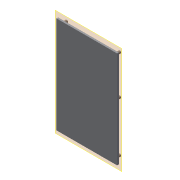
# Autodesk Inventor part: 200_Gearbox_conterplate
Saved by Autodesk Inventor 2019 (Build 230136000, 136)
## iProperties
Created: 2019-07-08
Part Number: 200_Gearbox_conterplate
Material: Generic
Document SubType Name: Modeling
Designer: diederichbenedict
Density: 1 g/cm^3
Appearance: Default
Author: diederichbenedict
Autodesk Inventor part; units mm, degrees
ref_plane "YZ Plane" through (0, 0, 0) normal (1, 0, 0) x (0, 1, 0)
ref_plane "XZ Plane" through (0, 0, 0) normal (0, 1, 0) x (-1, 0, 0)
ref_plane "XY Plane" through (0, 0, 0) normal (0, 0, 1) x (1, 0, 0)
ref_plane "Work Plane1" through (0, 0, 0) normal (0, 0, 1) x (1, 0, 0)
sketch "Sketch1" plane through (0, 0, 0) normal (0, 0, 1) x (1, 0, 0)
  circle A0 centre (-12.2447, -18.3325) radius 0.75 projected
  circle A1 centre (12.2447, 22.8412) radius 0.75 projected
  circle A2 centre (12.2447, 4.8925) radius 0.75 projected
  circle A3 centre (-12.2447, 4.8925) radius 0.75 projected
  circle A4 centre (12.2447, -18.3325) radius 0.75 projected
  circle A5 centre (-12.2447, 22.8412) radius 0.75 projected
  line L0 (-14, -20.0878) -> (14, -20.0878) projected
  line L1 (14, -20.0878) -> (14, 24.5965) projected
  line L2 (14, 24.5965) -> (8.6716, 24.5965) projected
  arc A6 (7.3084, 6.3656) -> (8.6716, 24.5965) centre (0, 16.0785) ccw projected
  line L3 (7.3084, 6.3656) -> (7.3084, 3.43) projected
  arc A7 (-7.3084, 3.43) -> (7.3084, 3.43) centre (0, -6.0878) ccw projected
  line L4 (-7.3084, 3.43) -> (-7.3084, 6.3656) projected
  arc A8 (-8.6716, 24.5965) -> (-7.3084, 6.3656) centre (0, 16.0785) ccw projected
  line L5 (-8.6716, 24.5965) -> (-14, 24.5965) projected
  line L6 (-14, 24.5965) -> (-14, -20.0878) projected
  line L7 (8.6716, 24.5965) -> (-8.6716, 24.5965)
  point P0 (0, 0)
  constraints: 2 end point, 1 horizontal
extrude "Extrusion1" add sketch "Sketch1" along normal blind 0.8 contours A0 | A1 | A2 | A3 | A4 | A5 | L6 L5 A8 L4 A7 L3 A6 L2 L1 L0 | L7 A6 L3 A7 L4 A8
sketch "Sketch2" plane through (0, 0, 0.8) normal (0, 0, 1) x (1, 0, 0)
  circle A0 centre (-12.2447, -18.3325) radius 0.75 construction
  circle A1 centre (12.2447, 22.8412) radius 0.75 construction
  circle A2 centre (12.2447, 4.8925) radius 0.75 construction
  circle A3 centre (-12.2447, 4.8925) radius 0.75 construction
  circle A4 centre (12.2447, -18.3325) radius 0.75 construction
  circle A5 centre (-12.2447, 22.8412) radius 0.75 construction
  circle A6 centre (0, -6.0878) radius 9.5 construction
  line L0 (14, -20.0878) -> (-14, -20.0878) construction
  line L1 (-14, -20.0878) -> (-14, 24.5965) construction
  line L2 (-14, 24.5965) -> (14, 24.5965) construction
  line L3 (14, 24.5965) -> (14, -20.0878) construction
  circle A7 centre (-12.2447, 22.8412) radius 0.6
  circle A8 centre (-12.2447, 4.8925) radius 0.6
  circle A9 centre (-12.2447, -18.3325) radius 0.6
  circle A10 centre (12.2447, -18.3325) radius 0.6
  circle A11 centre (12.2447, 4.8925) radius 0.6
  circle A12 centre (12.2447, 22.8412) radius 0.6
  dimension "a1" = 1.2
  dimension "d3" = 1.2
  dimension "d4" = 1.2
  dimension "d5" = 1.2
  dimension "d6" = 1.2
  dimension "d7" = 1.2
  constraints: 6 centre point, 6 coincident
  measures "a1" diameter of A7
  measures "d3" diameter of A8
  measures "d4" diameter of A9
  measures "d5" diameter of A10
  measures "d6" diameter of A11
  measures "d7" diameter of A12
extrude "Extrusion2" add sketch "Sketch2" against normal blind 3
equation "\"d3\" = a1"
equation "\"d4\" = a1"
equation "\"d5\" = a1"
equation "\"d6\" = a1"
equation "\"d7\" = a1"
body "Solid1"
